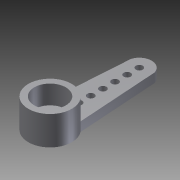
# Autodesk Inventor part: Servo_Arm
Saved by Autodesk Inventor 2011 SP2 (Build 150309200, 309)
## iProperties
Created: 2015-10-31
Part Number: Servo_Arm
Document SubType Name: Modeling
Designer: Ernest
Density: 1 g/cm^3
Author: Ernest
Autodesk Inventor part; units mm, degrees
ref_plane "YZ Plane" through (0, 0, 0) normal (1, 0, 0) x (0, 1, 0)
ref_plane "XZ Plane" through (0, 0, 0) normal (0, 1, 0) x (-1, 0, 0)
ref_plane "XY Plane" through (0, 0, 0) normal (0, 0, 1) x (1, 0, 0)
sketch "Sketch1" plane through (0, 0, 0) normal (0, 0, 1) x (1, 0, 0)
  circle A0 centre (0, 0) radius 3.45
  line L0 (0, 0) -> (14.75, 0) construction
  line L1 (14.75, 0) -> (14.75, 1.875) construction
  line L2 (14.75, 0) -> (14.75, -1.875) construction
  line L3 (14.75, 0) -> (16.15, 0) construction
  arc A1 (14.75, -1.875) -> (14.75, 1.875) centre (14.1944, 0) ccw
  line L4 (2.1159, 2.725) -> (2.1159, -2.725) construction
  line L5 (2.1159, 2.725) -> (14.75, 1.875)
  line L6 (2.1159, -2.725) -> (14.75, -1.875)
  circle A2 centre (14.1944, 0) radius 0.55
  circle A3 centre (4.5454, 0) radius 0.55
  circle A4 centre (6.4752, 0) radius 0.55
  circle A5 centre (8.405, 0) radius 0.55
  circle A6 centre (10.3348, 0) radius 0.55
  circle A7 centre (12.2646, 0) radius 0.55
  dimension "d0" = 6.9
  dimension "d1" = 14.75
  dimension "d2" = 1.875
  dimension "d3" = 1.875
  dimension "d4" = 1.4
  dimension "d5" = 5.45
  dimension "d12" = 1.1
  dimension "d13" = 1.1
  dimension "d14" = 1.1
  dimension "d15" = 1.1
  dimension "d16" = 1.1
  dimension "d17" = 1.1
  dimension "d18" = 1.9298
  dimension "d19" = 1.9298
  dimension "d20" = 1.9298
  dimension "d21" = 1.9298
  dimension "d22" = 1.9298
  constraints: 14 end point, 8 centre point, 5 point on circle, 5 point on line, 3 perpendicular, 2 coincident, 1 collinear, 1 horizontal
  measures "d0" diameter of A0
  measures "d1" distance of L0.start L0.end
  measures "d2" distance of L0.end L1.end
  measures "d3" distance of L0.end L2.end
  measures "d4" distance of L0.end L3.end
  measures "d5" distance of L4.start L4.end
  measures "d12" diameter of A2
  measures "d13" diameter of A3
  measures "d14" diameter of A4
  measures "d15" diameter of A5
  measures "d16" diameter of A6
  measures "d17" diameter of A7
  measures "d18" distance of A2.centre A7.centre
  measures "d19" distance of A6.centre A7.centre
  measures "d20" distance of A5.centre A6.centre
  measures "d21" distance of A4.centre A5.centre
  measures "d22" distance of A3.centre A4.centre
extrude "Extrusion1" add sketch "Sketch1" along normal blind 1.45 contours A0 L5 A1 L6
extrude "Extrusion2" add sketch "Sketch1" along normal blind 4.6 contours A0
sketch "Sketch2" plane through (0, 0, 0) normal (0, 0, -1) x (-1, 0, 0)
  arc A0 (-2.1159, -2.725) -> (-2.1159, 2.725) centre (0, 0) ccw projected
  circle A1 centre (0, 0) radius 1.175
  dimension "d27" = 2.35
  constraints: 1 centre point, 1 coincident
  measures "d27" diameter of A1
extrude "Extrusion3" cut sketch "Sketch2" against normal up to next
sketch "Sketch3" plane through (0, 0, 4.6) normal (0, 0, 1) x (1, 0, 0)
  circle A0 centre (0, 0) radius 1.175 projected
  circle A1 centre (0, 0) radius 3.45 projected
  circle A2 centre (0, 0) radius 2.5
  dimension "d30" = 5
  constraints: 1 centre point, 1 coincident
  measures "d30" diameter of A2
extrude "Extrusion4" cut sketch "Sketch3" against normal blind 3 contours A2
sketch "Sketch4" plane through (0, 0, 0) normal (0, 0, -1) x (-1, 0, 0)
  circle A0 centre (0, 0) radius 1.175 projected
  circle A1 centre (0, 0) radius 2.5 projected
  circle A2 centre (0, 0) radius 2.5 projected
  circle A3 centre (0, 0) radius 2.5
  constraints: 1 centre point, 1 coincident
extrude "Extrusion5" cut sketch "Sketch4" against normal blind 0.65
body "Solid1"
